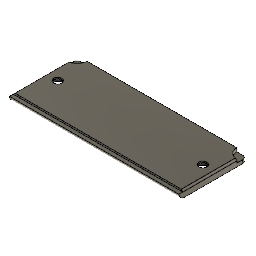
P3_Clean_Slate v3 (Autodesk Fusion 360 design; units mm, degrees)
Autodesk Fusion 360 part; units mm, degrees
sketch "草图1" plane through (0, 0, 0) normal (0, 0, 1) x (1, 0, 0)
  line L0 (0, 0) -> (43, 0)
  line L1 (43, 0) -> (43, 17.2)
  line L2 (43, 17.2) -> (0, 17.2)
  line L3 (0, 17.2) -> (0, 0)
  line L4 (0, 17.2) -> (3.1, 17.2) construction
  line L5 (3.1, 17.2) -> (3.1, 9.2) construction
  line L6 (3.1, 9.2) -> (0, 9.2) construction
  line L7 (0, 9.2) -> (0, 17.2) construction
  line L8 (21.5, 17.2) -> (21.5, 0) construction
  circle A0 centre (3.1, 9.2) radius 1.025
  circle A1 centre (3.1, 9.2) radius 2.05
  circle A2 centre (39.9, 9.2) radius 1.025
  circle A3 centre (39.9, 9.2) radius 2.05
  dimension "d1" = 43
  dimension "d2" = 17.2
  dimension "d17" = 3.1
  dimension "d18" = 8
  dimension "d19" = 2.05
  dimension "d20" = 4.1
  constraint horizontal L0
  constraint vertical L1
  constraint horizontal L2
  constraint vertical L3
  constraint coincident L0.start L3.end
  constraint horizontal L4
  constraint vertical L5
  constraint horizontal L6
  constraint vertical L7
  constraint midpoint L2 L8.start
  constraint midpoint L0 L8.end
  constraint coincident L5.end L6.start
  constraint concentric A0 A1
  constraint symmetric L8 A0 A2
  constraint symmetric L8 A1 A3
  measures "d1" distance of L0.start L0.end
  measures "d2" distance of L0.start L2.end
  measures "d17" distance of L2.end L4.end
  measures "d18" distance of L2.end L6.end
  measures "d19" diameter of A0
  measures "d20" diameter of A1
extrude "拉伸1" add sketch "草图1" along normal blind 1.8 contours L0 L1 L2 L3 | A0 | A1 | A2 | A3
sketch "草图2" plane through (0, 0, 1.8) normal (0, 0, 1) x (-1, 0, 0)
  line L0 (0, -17.2) -> (0, 0)
  line L1 (0, 0) -> (-43, 0)
  line L2 (-43, 0) -> (-43, -17.2)
  line L3 (-43, -17.2) -> (0, -17.2)
  circle A0 centre (0, -17.2) radius 2.5
  circle A1 centre (-43, -17.2) radius 2.5
  line L4 (0, 0) -> (-43, 0)
  line L5 (-43, 0) -> (-43, -1)
  line L6 (-43, -1) -> (0, -1)
  line L7 (0, -1) -> (0, 0)
  dimension "d5" = 5
  dimension "d6" = 5
  dimension "d11" = 1
  constraint coincident L0.start L3.end
  constraint coincident L2.end L3.start
  constraint horizontal L4
  constraint vertical L5
  constraint horizontal L6
  constraint vertical L7
  constraint coincident L0.end L1.start
  measures "d5" diameter of A0
  measures "d6" diameter of A1
  measures "d11" distance of L0.end L6.end
extrude "拉伸2" cut sketch "草图2" against normal blind 0.9 contours L0 L3 A0 | L2 L3 A1 picked at (-1.3308, -16.2037) picked at (-41.5409, -16.4033)
fillet "圆角1" radius 1 2 edges at (43, 17.2, 0.45) (0, 17.2, 0.45)
extrude "拉伸3" cut sketch "草图2" against normal blind 0.4 contours L0 L1 L2 L4 L5 L6 L7
fillet "圆角3" radius 1.5 1 edges at (21.5, 0, 0)
chamfer "倒角1" distance 0.4 angle 45 2 edges at (43, 7.85, 1.8) (0, 7.85, 1.8)
extrude "拉伸4" cut sketch "草图1" along normal up to surface (1.8 mm away) contours A0 | A2
extrude "拉伸5" cut sketch "草图1" along normal blind 0.5 contours A1 | A3
chamfer "倒角3" distance 1 angle 45 2 edges at (38.9444, 9.5707, 0.5) (2.1444, 9.5707, 0.5)
chamfer "倒角4" distance 0.2 angle 45 2 edges at (1.1887, 8.4587, 0) (37.9887, 8.4587, 0)
named bodies: "P3_Panel"
